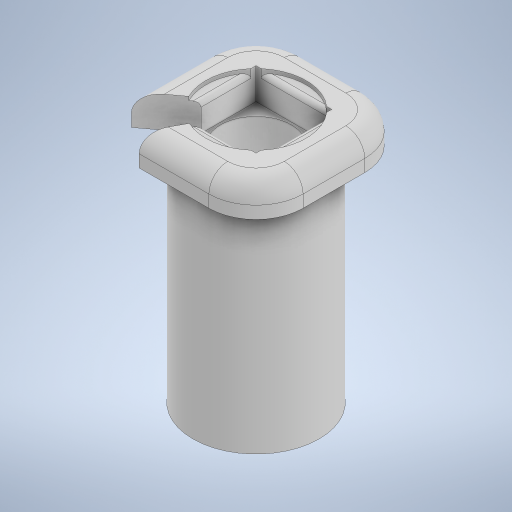
# Autodesk Inventor part: Wheel Adaptor
Saved by Autodesk Inventor 2024.2 (Build 282272000, 272)
## iProperties
Created: 2023-12-29
Part Number: Wheel Adaptor
Material: Generic
Document SubType Name: Modeling
Designer: R730
Density: 1 g/cm^3
Appearance: Default
Author: R730
Autodesk Inventor part; units mm, degrees
ref_plane "YZ Plane" through (0, 0, 0) normal (1, 0, 0) x (0, 1, 0)
ref_plane "XZ Plane" through (0, 0, 0) normal (0, 1, 0) x (-1, 0, 0)
ref_plane "XY Plane" through (0, 0, 0) normal (0, 0, 1) x (1, 0, 0)
sketch "Sketch2" plane through (0, 0, 0) normal (0, 1, 0) x (-1, 0, 0)
  line L0 (21, 21) -> (-21, 21)
  line L1 (-21, 21) -> (-21, -21)
  line L2 (-21, -21) -> (21, -21)
  line L3 (21, -21) -> (21, 21)
  line L4 (21, 21) -> (-21, -21) construction
  line L5 (-21, 21) -> (21, -21) construction
  point P0 (0, 0)
  point P1 (-21, 0)
  dimension "d1" = 42
  dimension "d2" = 42
  constraints: 12 end point, 3 midpoint, 2 parallel, 1 horizontal, 1 perpendicular
  measures "d1" distance from line of point (-21, 0) L3
  measures "d2" distance between parallel lines of L0 L2
extrude "Extrusion1" add sketch "Sketch2" along normal blind 7.4
sketch "Sketch3" plane through (0, 7.4, 0) normal (0, 1, 0) x (1, 0, 0)
  line L0 (-10.2, -10.2) -> (10.2, -10.2)
  line L1 (10.2, -10.2) -> (10.2, 10.2)
  line L2 (10.2, 10.2) -> (-10.2, 10.2)
  line L3 (-10.2, 10.2) -> (-10.2, -10.2)
  line L4 (-10.2, -10.2) -> (10.2, 10.2) construction
  line L5 (10.2, -10.2) -> (-10.2, 10.2) construction
  line L6 (-4.612, -10.2) -> (-10.4855, -21)
  line L7 (-10.2, -4.5965) -> (-21, -12.5849)
  line L8 (-21, 21) -> (-21, -21) projected
  line L9 (-21, -12.5849) -> (-21, -21)
  line L10 (-21, -21) -> (-10.4855, -21)
  line L11 (-21, -21) -> (21, -21) projected
  line L12 (-10.2, -10.2) -> (-10.2, -4.5965)
  point P0 (0, 0)
  dimension "d5" = 20.4
  dimension "d6" = 20.4
  dimension "d9" = 5.588
  constraints: 22 end point, 3 point on line, 2 collinear, 2 midpoint, 2 parallel, 1 horizontal, 1 perpendicular, 1 vertical
  measures "d5" distance of L2.end L1.end
  measures "d6" distance between parallel lines of L0 L2
  measures "d9" distance of L0.start L6.start
extrude "Extrusion2" cut sketch "Sketch3" against normal blind 7.4
sketch "Sketch4" plane through (0, 7.4, 0) normal (0, 1, 0) x (1, 0, 0)
  circle A0 centre (0, 0) radius 13.5
  line L0 (-10.2, -4.5965) -> (-21, -12.5849) projected
  line L1 (-12.0945, -5.9978) -> (-21, -12.5849)
  line L2 (-21, -12.5849) -> (-21, 21)
  line L3 (-21, 21) -> (21, 21)
  line L4 (21, 21) -> (21, -21.0478)
  line L5 (-4.612, -10.2) -> (-10.4855, -21) projected
  line L6 (-5.7161, -12.2301) -> (-10.4855, -21)
  line L7 (-10.4855, -21) -> (21, -21) projected
  line L8 (21, -21) -> (-10.4855, -21)
  line L9 (10.2, 10.2) -> (10.2, -10.2) projected
  line L10 (8.8436, -10.2) -> (10.2, -10.2)
  line L11 (10.2, -10.2) -> (10.2, -8.8436)
  line L12 (-10.2, 10.2) -> (10.2, 10.2) projected
  line L13 (8.8436, 10.2) -> (10.2, 10.2)
  line L14 (10.2, 10.2) -> (10.2, 8.8436)
  line L15 (-10.2, -4.5965) -> (-10.2, 10.2) projected
  line L16 (-10.2, 8.8436) -> (-10.2, 10.2)
  line L17 (-10.2, 10.2) -> (-8.8436, 10.2)
  point P0 (-8.8436, 10.2)
  point P1 (10.2, -8.8436)
  dimension "d10" = 27
  constraints: 24 end point, 6 point on line, 4 collinear, 3 perpendicular, 1 coincident, 1 horizontal, 1 vertical, 10 other
extrude "Extrusion3" add sketch "Sketch4" along normal blind 1 contours A0 L9 L12 L15 L0 L2 L3 L4 L7 L5 L10
fillet "Fillet4" radius 12.7 3 edges at (21, 4.2, 21) (21, 4.2, -21) (-21, 4.2, -21)
fillet "Fillet5" radius 5.08 7 edges at (-1.0927, 8.4, 21) (21, 8.4, 0) (17.2803, 8.4, -17.2803) (0, 8.4, -21) (-17.2803, 8.4, -17.2803) (-21, 8.4, 2.1424) (17.2803, 8.4, 17.2803)
fillet "Fillet6" radius 1.27 4 edges at (2.1158, 7.4, 10.2) (-10.2, 7.4, -2.1236) (0, 7.4, -10.2) (10.2, 7.4, 0)
sketch "Sketch5" plane through (0, 0, 0) normal (0, -1, 0) x (1, 0, 0)
  circle A0 centre (0, 0) radius 17
  circle A1 centre (0, 0) radius 9.6
  dimension "d19" = 34
  dimension "d20" = 19.2
  constraints: 2 centre point, 2 coincident
  measures "d19" diameter of A0
  measures "d20" diameter of A1
extrude "Extrusion4" add sketch "Sketch5" along normal blind 13
sketch "Sketch6" plane through (0, -13, 0) normal (0, -1, 0) x (1, 0, 0)
  circle A0 centre (0, 0) radius 17
  circle A1 centre (0, 0) radius 6.5
  dimension "d23" = 13
  constraints: 2 centre point, 2 coincident
  measures "d23" diameter of A1
extrude "Extrusion5" add sketch "Sketch6" along normal blind 15
sketch "Sketch8" plane through (0, -28, 0) normal (0, -1, 0) x (1, 0, 0)
  circle A0 centre (0, 0) radius 17
  circle A1 centre (0, 0) radius 3
  dimension "d29" = 6
  dimension "d32" = 34
  constraints: 2 centre point, 2 coincident
  measures "d29" diameter of A1
  measures "d32" diameter of A0
extrude "Extrusion7" add sketch "Sketch8" along normal blind 32
body "Solid1"
